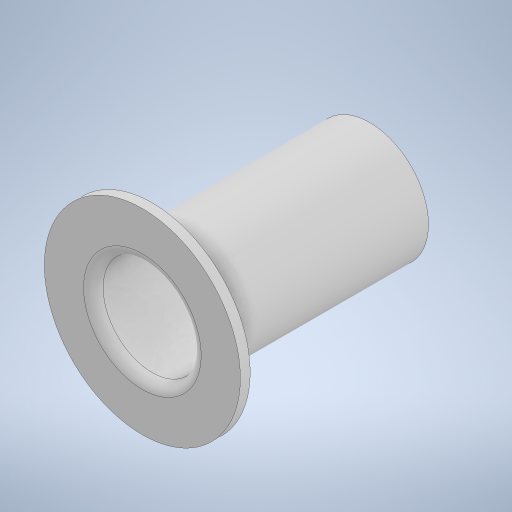
# Autodesk Inventor part: Standard Servo Brass Sleeve
Saved by Autodesk Inventor 2023 (Build 270158000, 158)
## iProperties
Created: 2023-09-05
Part Number: Standard Servo Brass Sleeve
Material: Generic
Document SubType Name: Modeling
Designer: Nate
Density: 1 g/cm^3
Appearance: Default
Author: Nate
Autodesk Inventor part; units mm, degrees
ref_plane "YZ Plane" through (0, 0, 0) normal (1, 0, 0) x (0, 1, 0)
ref_plane "XZ Plane" through (0, 0, 0) normal (0, 1, 0) x (-1, 0, 0)
ref_plane "XY Plane" through (0, 0, 0) normal (0, 0, 1) x (1, 0, 0)
sketch "Sketch1" plane through (0, 0, 0) normal (0, 0, 1) x (1, 0, 0)
  circle A0 centre (0, 0) radius 2.5
  circle A1 centre (0, 0) radius 1.25
  circle A2 centre (0, 0) radius 1.5
  dimension "d0" = 5
  dimension "d1" = 2.5
  dimension "d2" = 3
  constraints: 3 centre point, 3 coincident
  measures "d0" diameter of A0
  measures "d1" diameter of A1
  measures "d2" diameter of A2
extrude "Extrusion1" add sketch "Sketch1" against normal blind 0.25 contours A0
extrude "Extrusion2" add sketch "Sketch1" against normal blind 5.8 contours A2
fillet "Fillet1" radius 0.25 1 edges at (-1.25, 0, 0)
fillet "Fillet2" radius 0.25 1 edges at (-1.5, 0, -0.25)
body "Solid1"
